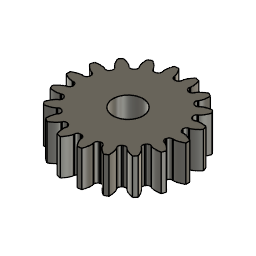
PinionGear (Autodesk Fusion 360 design; units mm, degrees)
part number: 2026-05-31-22-59-23-955
description: Spur Gear; Module: 0.5; Num Teeth: 18; Pressure Angle: 20.0; Backlash: 0.00 mm
part number: 2026-05-31-23-23-50-884
Autodesk Fusion 360 part; units mm, degrees
sketch "Base Circle" plane through (0, 0, 0) normal (0, 0, 1) x (1, 0, 0) in component "Spur Gear 18 teeth"
  circle A0 centre (0, 0) radius 3.9215
  circle A1 centre (0, 0) radius 1.25
extrude "Extrude1" add sketch "Base Circle" along normal blind 10 in component "Spur Gear 18 teeth"
sketch "Gear Tooth" plane through (0, 0, 0) normal (0, 0, 1) x (1, 0, 0) in component "Spur Gear 18 teeth"
  spline S0 degree 5 poles (4.2066, -0.4313) (4.2088, -0.4315) (4.2132, -0.4319) (4.2199, -0.4323) (4.2289, -0.4325) (4.2401, -0.4323) (4.2513, -0.4317) (4.2626, -0.431) (4.2739, -0.43) (4.2851, -0.4291) (4.2964, -0.428) (4.3077, -0.4268) (4.319, -0.4255) (4.3303, -0.424) (4.3416, -0.4224) (4.353, -0.4206) (4.3643, -0.4186) (4.3757, -0.4166) (4.387, -0.4144) (4.3983, -0.4122) (4.4097, -0.4098) (4.421, -0.4074) (4.4324, -0.4048) (4.4438, -0.4022) (4.4551, -0.3994) (4.4665, -0.3965) (4.4779, -0.3936) (4.4892, -0.3905) (4.5006, -0.3874) (4.512, -0.3841) (4.5233, -0.3808) (4.5347, -0.3774) (4.5461, -0.3739) (4.5574, -0.3703) (4.5688, -0.3666) (4.5801, -0.3629) (4.5915, -0.359) (4.6029, -0.3551) (4.6142, -0.3511) (4.6256, -0.347) (4.6369, -0.3428) (4.6483, -0.3386) (4.6596, -0.3343) (4.671, -0.3299) (4.6823, -0.3254) (4.6936, -0.3208) (4.705, -0.3162) (4.7163, -0.3115) (4.7276, -0.3067) (4.7389, -0.3018) (4.7502, -0.2969) (4.7615, -0.2919) (4.7728, -0.2868) (4.7841, -0.2817) (4.7954, -0.2764) (4.8067, -0.2711) (4.8179, -0.2658) (4.8292, -0.2603) (4.8404, -0.2548) (4.8517, -0.2492) (4.8629, -0.2436) (4.8742, -0.2378) (4.8854, -0.232) (4.8966, -0.2262) (4.9078, -0.2203) (4.919, -0.2143) (4.9302, -0.2082) (4.9414, -0.2021) (4.9525, -0.1959) (4.9637, -0.1896) (4.9748, -0.1833) (4.9837, -0.1781) (4.9904, -0.1743) (4.9949, -0.1717) (4.9971, -0.1704) knots 0 0 0 0 0 0 0.01428571 0.02857143 0.04285714 0.05714286 0.07142857 0.08571429 0.1 0.11428571 0.12857143 0.14285714 0.15714286 0.17142857 0.18571429 0.2 0.21428571 0.22857143 0.24285714 0.25714286 0.27142857 0.28571429 0.3 0.31428571 0.32857143 0.34285714 0.35714286 0.37142857 0.38571429 0.4 0.41428571 0.42857143 0.44285714 0.45714286 0.47142857 0.48571429 0.5 0.51428571 0.52857143 0.54285714 0.55714286 0.57142857 0.58571429 0.6 0.61428571 0.62857143 0.64285714 0.65714286 0.67142857 0.68571429 0.7 0.71428571 0.72857143 0.74285714 0.75714286 0.77142857 0.78571429 0.8 0.81428571 0.82857143 0.84285714 0.85714286 0.87142857 0.88571429 0.9 0.91428571 0.92857143 0.94285714 0.95714286 0.97142857 0.98571429 1 1 1 1 1 1
  spline S1 degree 5 poles (4.2066, 0.4313) (4.2088, 0.4315) (4.2132, 0.4319) (4.2199, 0.4323) (4.2289, 0.4325) (4.2401, 0.4323) (4.2513, 0.4317) (4.2626, 0.431) (4.2739, 0.43) (4.2851, 0.4291) (4.2964, 0.428) (4.3077, 0.4268) (4.319, 0.4255) (4.3303, 0.424) (4.3416, 0.4224) (4.353, 0.4206) (4.3643, 0.4186) (4.3757, 0.4166) (4.387, 0.4144) (4.3983, 0.4122) (4.4097, 0.4098) (4.421, 0.4074) (4.4324, 0.4048) (4.4438, 0.4022) (4.4551, 0.3994) (4.4665, 0.3965) (4.4779, 0.3936) (4.4892, 0.3905) (4.5006, 0.3874) (4.512, 0.3841) (4.5233, 0.3808) (4.5347, 0.3774) (4.5461, 0.3739) (4.5574, 0.3703) (4.5688, 0.3666) (4.5801, 0.3629) (4.5915, 0.359) (4.6029, 0.3551) (4.6142, 0.3511) (4.6256, 0.347) (4.6369, 0.3428) (4.6483, 0.3386) (4.6596, 0.3343) (4.671, 0.3299) (4.6823, 0.3254) (4.6936, 0.3208) (4.705, 0.3162) (4.7163, 0.3115) (4.7276, 0.3067) (4.7389, 0.3018) (4.7502, 0.2969) (4.7615, 0.2919) (4.7728, 0.2868) (4.7841, 0.2817) (4.7954, 0.2764) (4.8067, 0.2711) (4.8179, 0.2658) (4.8292, 0.2603) (4.8404, 0.2548) (4.8517, 0.2492) (4.8629, 0.2436) (4.8742, 0.2378) (4.8854, 0.232) (4.8966, 0.2262) (4.9078, 0.2203) (4.919, 0.2143) (4.9302, 0.2082) (4.9414, 0.2021) (4.9525, 0.1959) (4.9637, 0.1896) (4.9748, 0.1833) (4.9837, 0.1781) (4.9904, 0.1743) (4.9949, 0.1717) (4.9971, 0.1704) knots 0 0 0 0 0 0 0.01428571 0.02857143 0.04285714 0.05714286 0.07142857 0.08571429 0.1 0.11428571 0.12857143 0.14285714 0.15714286 0.17142857 0.18571429 0.2 0.21428571 0.22857143 0.24285714 0.25714286 0.27142857 0.28571429 0.3 0.31428571 0.32857143 0.34285714 0.35714286 0.37142857 0.38571429 0.4 0.41428571 0.42857143 0.44285714 0.45714286 0.47142857 0.48571429 0.5 0.51428571 0.52857143 0.54285714 0.55714286 0.57142857 0.58571429 0.6 0.61428571 0.62857143 0.64285714 0.65714286 0.67142857 0.68571429 0.7 0.71428571 0.72857143 0.74285714 0.75714286 0.77142857 0.78571429 0.8 0.81428571 0.82857143 0.84285714 0.85714286 0.87142857 0.88571429 0.9 0.91428571 0.92857143 0.94285714 0.95714286 0.97142857 0.98571429 1 1 1 1 1 1
  arc A0 (4.9971, -0.1704) -> (4.9971, 0.1704) centre (0, 0) ccw
  line L0 (3.8911, -0.3989) -> (4.2066, -0.4313)
  line L1 (3.8911, 0.3989) -> (4.2066, 0.4313)
  line L2 (3.8911, -0.3989) -> (3.8911, 0.3989)
  point P0 (4.262, -0.431)
  point P1 (4.3179, -0.4256)
  point P2 (4.3741, -0.4168)
  point P3 (4.4305, -0.4052)
  point P4 (4.4871, -0.3911)
  point P5 (4.5438, -0.3746)
  point P6 (4.6006, -0.3559)
  point P7 (4.6574, -0.3351)
  point P8 (4.7142, -0.3123)
  point P9 (4.7709, -0.2876)
  point P10 (4.8277, -0.261)
  point P11 (4.8843, -0.2326)
  point P12 (4.9408, -0.2024)
  point P13 (4.262, 0.431)
  point P14 (4.3179, 0.4256)
  point P15 (4.3741, 0.4168)
  point P16 (4.4305, 0.4052)
  point P17 (4.4871, 0.3911)
  point P18 (4.5438, 0.3746)
  point P19 (4.6006, 0.3559)
  point P20 (4.6574, 0.3351)
  point P21 (4.7142, 0.3123)
  point P22 (4.7709, 0.2876)
  point P23 (4.8277, 0.261)
  point P24 (4.8843, 0.2326)
  point P25 (4.9408, 0.2024)
extrude "Extrude2" add sketch "Gear Tooth" along normal blind 10 in component "Spur Gear 18 teeth"
fillet "Fillet1" radius 0.25 2 edges at (3.901, -0.4, 5) (3.901, 0.4, 5) in component "Spur Gear 18 teeth"
pattern_circular "C-Pattern1" count 18 over 360 about axis through (0, 0, 0) along (0, 0, 1) of "Extrude2", "Fillet1" in component "Spur Gear 18 teeth"
sketch "Diametrial Pitch Circle" plane through (0, 0, 0) normal (0, 0, 1) x (1, 0, 0) in component "Spur Gear 18 teeth"
  circle A0 centre (0, 0) radius 4.5 construction
extrude "Extrude3" cut 1 faces at (3.0102, 0, 10) along direction (0, 0, -1) blind 7 in component "Spur Gear 18 teeth"
component "Spur Gear 18 teeth" placed x (1, 0, 0) y (0, 1, 0) z (0, 0, 1) at (0, 0, 0)
